Autodesk Fusion 360 part; units mm, degrees
(part 2 of 2)
sketch "Sketch20" plane through (0, 8, 0) normal (0, 1, 0) x (-1, 0, 0)
  line L0 (-15, 29) -> (-15, 41)
  line L1 (-15, 41) -> (-16, 41)
  line L2 (-16, 41) -> (-16, 29)
  line L3 (-16, 29) -> (-15, 29)
  line L4 (-16, 41) -> (-15, 41)
  line L5 (-15, 29) -> (-15, 41)
  line L6 (-15, 29) -> (-16, 29)
  line L7 (-16, 29) -> (-16, 41)
  line L8 (-16, 41) -> (-16, 44)
  line L9 (-16, 44) -> (-12, 44)
  line L10 (-12, 44) -> (-12, 26)
  line L11 (-12, 26) -> (-16, 26)
  line L12 (-16, 26) -> (-16, 29)
  constraint coincident L1.end L2.start
  constraint coincident L0.end L1.start
  constraint coincident L0.start L3.end
  constraint coincident L2.end L3.start
  constraint perpendicular L1 L8
  constraint perpendicular L2 L9
  constraint perpendicular L9 L10
  constraint perpendicular L10 L11
  constraint perpendicular L6 L12
extrude "Extrude78" cut sketch "Sketch20" against normal blind 6.5 contours L0 L1 L3 L4 L5 L6 L8 L9 L10 L11 L12 bodies 1
extrude "Extrude79" add 1 faces at (15, 5.8333, 33) along direction (-1, 0, 0) blind 1 on bodies 1 bodies 1
fillet "Fillet28" radius 3 3 edges at (15, 1.5, 41) (14, 1.5, 35) (15, 1.5, 29) on bodies 1
sketch "Sketch21" plane through (14, 0, 0) normal (-1, 0, 0) x (0, -1, 0)
  line L0 (-4.5, 29) -> (-4.5, 41)
  line L1 (-4.5, 41) -> (-8, 41)
  line L2 (-8, 41) -> (-8, 29)
  line L3 (-8, 29) -> (-4.5, 29)
extrude "Extrude80" add 1 faces at (14.6667, 8, 37) along direction (0, 1, 0) blind 1 on bodies 1 bodies 1
extrude "Extrude81" add 1 faces at (15.3333, -8, 37) along direction (0, -1, 0) blind 1 on bodies 1 bodies 1
sketch "Sketch22" plane through (14, 0, 0) normal (-1, 0, 0) x (0, -1, 0)
  line L0 (-4.5, 29) -> (-4.5, 41)
  line L1 (-4.5, 41) -> (-9, 41)
  line L2 (-9, 41) -> (-9, 29)
  line L3 (-9, 29) -> (-4.5, 29)
  line L4 (-9, 41) -> (-7, 41)
  line L5 (-9, 29) -> (-7, 29)
  line L6 (-7, 29) -> (-7, 41)
  line L7 (-9, 41) -> (-9, 29)
  dimension "d368" = 2
  dimension "d369" = 2
  constraint coincident L1.end L2.start
  constraint perpendicular L2 L4
  constraint coincident L2.end L3.start
  constraint perpendicular L2 L5
  measures "d368" distance of L1.end L4.end
  measures "d369" distance of L2.end L5.end
extrude "Extrude82" add sketch "Sketch22" along normal blind 4 contours L1 L2 L3 L4 L5 L6 L7 bodies 1
sketch "Sketch23" plane through (15, 0, 0) normal (-1, 0, 0) x (0, -1, 0)
  line L0 (9, 41) -> (4.5, 41)
  arc A0 (2.5, 41.7639) -> (4.5, 41) centre (4.5, 44) ccw
  line L1 (2.5, 41.7639) -> (2.5, 28.2361)
  arc A1 (4.5, 29) -> (2.5, 28.2361) centre (4.5, 26) ccw
  line L2 (4.5, 29) -> (9, 29)
  line L3 (9, 29) -> (9, 41)
  line L4 (9, 41) -> (7, 41)
  line L5 (7, 41) -> (7, 29)
  line L6 (7, 29) -> (9, 29)
  line L7 (9, 29) -> (9, 41)
  dimension "d372" = 2
  constraint horizontal L4
  constraint vertical L5
  constraint horizontal L6
  constraint vertical L7
  constraint coincident L0.start L3.end
  measures "d372" distance of L0.start L4.end
extrude "Extrude83" add sketch "Sketch23" along normal blind 4 contours L0 L2 L3 L4 L5 L6 L7 bodies 1
fillet "Fillet29" radius 1 1 edges at (14, 7, 35) on bodies 1
fillet "Fillet30" radius 1 1 edges at (15, -7, 35) on bodies 1
fillet "Fillet31" radius 2 2 edges at (16, 9, 35) (16, -9, 35) on bodies 1
fillet "Fillet32" radius 3 2 edges at (16, 0, 65) (16, 0, 5) on bodies 1
fillet "Fillet33" radius 1 4 edges at (10, 7, 35) (10, 9, 35) (10, 8, 41) (10, 8, 29) on bodies 1
fillet "Fillet34" radius 1 4 edges at (11, -9, 35) (11, -8, 41) (11, -7, 35) (11, -8, 29) on bodies 1
